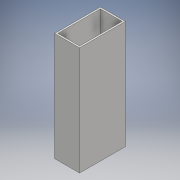
# Autodesk Inventor part: LiFeGuard
Saved by Autodesk Inventor 2018 (Build 220112000, 112)
## iProperties
Created: 2018-08-27
Part Number: LiFeGuard
Material: 一般
Document SubType Name: Modeling
Designer: shun2
Density: 1 g/cm^3
Appearance: 既定
Author: shun2
Autodesk Inventor part; units mm, degrees
ref_plane "YZ Plane" through (0, 0, 0) normal (1, 0, 0) x (0, 1, 0)
ref_plane "XZ Plane" through (0, 0, 0) normal (0, 1, 0) x (-1, 0, 0)
ref_plane "XY Plane" through (0, 0, 0) normal (0, 0, 1) x (1, 0, 0)
sketch "スケッチ1" plane through (0, 0, 0) normal (0, 0, 1) x (1, 0, 0)
  line L0 (0, 0) -> (30, 0)
  line L1 (30, 0) -> (30, 55)
  line L2 (30, 55) -> (0, 55)
  line L3 (0, 55) -> (0, 2)
  line L4 (2, 53) -> (2, 2)
  line L5 (2, 2) -> (28, 2)
  line L6 (28, 53) -> (28, 2)
  line L7 (2, 53) -> (28, 53)
  line L8 (0, 2) -> (0, 0)
  dimension "d0" = 30
  dimension "d1" = 55
  constraints: 18 end point, 5 perpendicular, 2 parallel, 1 horizontal, 1 vertical
  measures "d0" distance of L2.end L1.end
  measures "d1" distance of L1.end L0.end
extrude "押し出し1" add sketch "スケッチ1" along normal blind 130
